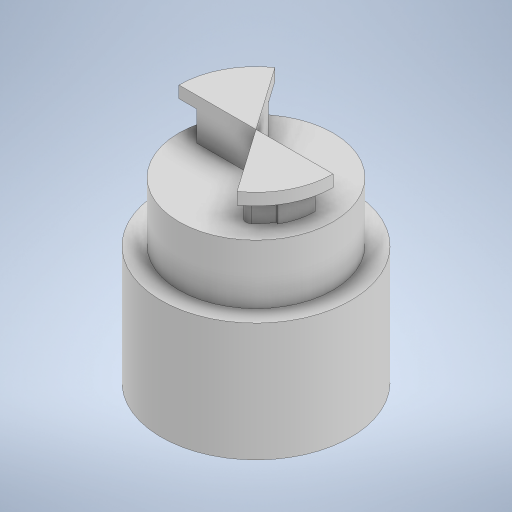
# Autodesk Inventor part: kumi4-1
Saved by Autodesk Inventor 2023.2 (Build 272271000, 271)
## iProperties
Created: 2022-12-20
Part Number: kumi4-1
Material: 一般
Document SubType Name: Modeling
Designer: 千葉 俊輔
Density: 1 g/cm^3
Appearance: 既定
Author: 千葉 俊輔
Autodesk Inventor part; units mm, degrees
ref_plane "YZ Plane" through (0, 0, 0) normal (1, 0, 0) x (0, 1, 0)
ref_plane "XZ Plane" through (0, 0, 0) normal (0, 1, 0) x (-1, 0, 0)
ref_plane "XY Plane" through (0, 0, 0) normal (0, 0, 1) x (1, 0, 0)
sketch "スケッチ1" plane through (0, 0, 0) normal (0, 1, 0) x (-1, 0, 0)
  circle A0 centre (0, 0) radius 16
  dimension "d0" = 32
  constraints: 1 centre point, 1 coincident
  measures "d0" diameter of A0
extrude "押し出し1" add sketch "スケッチ1" along normal blind 20
sketch "スケッチ2" plane through (0, 20, 0) normal (0, 1, 0) x (1, 0, 0)
  circle A0 centre (0, 0) radius 13
  dimension "d3" = 26
  constraints: 1 centre point, 1 coincident
  measures "d3" diameter of A0
extrude "押し出し2" add sketch "スケッチ2" along normal blind 10
sketch "スケッチ3" plane through (0, 30, 0) normal (0, 1, 0) x (1, 0, 0)
  arc A0 (-8.6603, 5) -> (-10, 0) centre (0, 0) ccw
  line L0 (0, 0) -> (-8.6603, 5) construction
  line L1 (0, 0) -> (-10, 0) construction
  arc A1 (-5.5063, 7.8639) -> (-8.3138, 4.8) centre (0, 0) ccw
  line L2 (0, 0) -> (-5.5063, 7.8639) construction
  line L3 (0, 0) -> (-8.3138, 4.8) construction
  arc A2 (8.6603, -5) -> (10, 0) centre (0, 0) ccw
  line L4 (0, 0) -> (8.6603, -5) construction
  line L5 (0, 0) -> (10, 0) construction
  arc A3 (5.5063, -7.8639) -> (8.3138, -4.8) centre (0, 0) ccw
  line L6 (0, 0) -> (5.5063, -7.8639) construction
  line L7 (0, 0) -> (8.3138, -4.8) construction
  line L8 (-8.6603, 5) -> (-8.3138, 4.8)
  line L9 (8.6603, -5) -> (8.3138, -4.8)
  line L10 (-5.5063, 7.8639) -> (5.5063, -7.8639)
  line L11 (-10, 0) -> (10, 0)
  dimension "d6" = 10
  dimension "d7" = 30
  dimension "d10" = 9.6
  dimension "d11" = 25
  dimension "d12" = 10
  dimension "d13" = 30
  dimension "d14" = 9.6
  dimension "d15" = 25
  constraints: 24 end point, 8 point on circle, 4 centre point, 4 coincident, 3 collinear, 2 point on line, 1 horizontal
  measures "d6" radius of A0
  measures "d7" angle of L0 L1
  measures "d10" radius of A1
  measures "d11" angle of L2 L3
  measures "d12" radius of A2
  measures "d13" angle of L4 L5
  measures "d14" radius of A3
  measures "d15" angle of L6 L7
extrude "押し出し3" add sketch "スケッチ3" along normal blind 5
fillet "フィレット1" radius 1 2 edges at (-5.5063, 32.5, -7.8639) (5.5063, 32.5, 7.8639)
sketch "スケッチ4" plane through (0, 35, 0) normal (0, 1, 0) x (1, 0, 0)
  line L0 (-4.8993, 6.9969) -> (0, 0) projected
  line L1 (4.8993, -6.9969) -> (0, 0) projected
  arc A0 (7.4565, -10.649) -> (13, 0) centre (0, 0) ccw
  line L2 (0, 0) -> (7.4565, -10.649) construction
  line L3 (0, 0) -> (13, 0) construction
  line L4 (0, 0) -> (10, 0) projected
  arc A1 (-7.4565, 10.649) -> (-13, 0) centre (0, 0) ccw
  line L5 (0, 0) -> (-7.4565, 10.649) construction
  line L6 (0, 0) -> (-13, 0) construction
  circle A2 centre (0, 0) radius 13 projected
  line L7 (7.4565, -10.649) -> (0, 0)
  line L8 (0, 0) -> (13, 0)
  line L9 (0, 0) -> (-13, 0)
  line L10 (0, 0) -> (-7.4565, 10.649)
  dimension "d21" = 13
  dimension "d22" = 55
  dimension "d23" = 13
  dimension "d24" = 55
  constraints: 16 end point, 4 point on circle, 3 collinear, 2 centre point, 2 coincident, 1 horizontal
  measures "d21" radius of A0
  measures "d22" angle of L2 L3
  measures "d23" radius of A1
  measures "d24" angle of L5 L6
extrude "押し出し4" add sketch "スケッチ4" along normal blind 2 contours L0 L9 A1 L10 | L4 L8 A0 L7 L1
